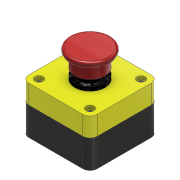
# Autodesk Inventor part: E-Stop
Saved by Autodesk Inventor 2022 (Build 260153000, 153)
## iProperties
Created: 2016-03-20
Part Number: E-Stop
Material: Generic
Document SubType Name: Modeling
Designer: Administrator
Density: 1 g/cm^3
Appearance: Default
Author: Administrator
Autodesk Inventor part; units mm, degrees
ref_plane "YZ Plane" through (0, 0, 0) normal (1, 0, 0) x (0, 1, 0)
ref_plane "XZ Plane" through (0, 0, 0) normal (0, 1, 0) x (-1, 0, 0)
ref_plane "XY Plane" through (0, 0, 0) normal (0, 0, 1) x (1, 0, 0)
sketch "Sketch1" plane through (0, 0, 0) normal (0, 0, 1) x (1, 0, 0)
  line L0 (-34, 34) -> (34, 34)
  line L1 (34, 34) -> (34, -34)
  line L2 (34, -34) -> (-34, -34)
  line L3 (-34, -34) -> (-34, 34)
  point P0 (0, 0)
  dimension "d0" = 34
  dimension "d1" = 34
  dimension "d2" = 34
  dimension "d3" = 34
  constraints: 8 end point, 2 parallel, 1 horizontal, 1 perpendicular
  measures "d0" distance from line of L3 point (0, 0)
  measures "d1" distance from line of L2 point (0, 0)
  measures "d2" distance from line of L1 point (0, 0)
  measures "d3" distance from line of L0 point (0, 0)
extrude "Extrusion1" add sketch "Sketch1" along normal blind 19
sketch "Sketch2" plane through (0, 0, 19) normal (0, 0, 1) x (1, 0, 0)
  circle A0 centre (0, 0) radius 15
  dimension "d6" = 30
  constraints: 1 centre point, 1 coincident
  measures "d6" diameter of A0
extrude "Extrusion2" add sketch "Sketch2" along normal blind 4
sketch "Sketch3" plane through (0, 0, 23) normal (0, 0, 1) x (1, 0, 0)
  circle A0 centre (0, 0) radius 11.25
  dimension "d9" = 22.5
  constraints: 1 centre point, 1 coincident
  measures "d9" diameter of A0
extrude "Extrusion3" add sketch "Sketch3" along normal blind 6
sketch "Sketch4" plane through (0, 0, 29) normal (0, 0, 1) x (1, 0, 0)
  circle A0 centre (0, 0) radius 15
  dimension "d12" = 30
  constraints: 1 centre point, 1 coincident
  measures "d12" diameter of A0
extrude "Extrusion4" add sketch "Sketch4" along normal blind 12
sketch "Sketch5" plane through (0, 0, 41) normal (0, 0, 1) x (1, 0, 0)
  circle A0 centre (0, 0) radius 20
  dimension "d15" = 40
  constraints: 1 centre point, 1 coincident
  measures "d15" diameter of A0
extrude "Extrusion5" add sketch "Sketch5" along normal blind 6
fillet "Fillet1" radius 2 1 edges at (-20, 0, 47)
fillet "Fillet2" radius 3 1 edges at (-20, 0, 41)
fillet "Fillet3" radius 7 4 edges at (34, 34, 9.5) (-34, 34, 9.5) (34, -34, 9.5) (-34, -34, 9.5)
sketch "Sketch6" plane through (0, 0, 0) normal (0, 0, -1) x (-1, 0, 0)
  arc A0 (-27, 34) -> (-34, 27) centre (-27, 27) ccw projected
  arc A1 (27, -34) -> (34, -27) centre (27, -27) ccw projected
  line L0 (-27, 27) -> (27, -27)
  arc A2 (34, 27) -> (27, 34) centre (27, 27) ccw projected
  arc A3 (-34, -27) -> (-27, -34) centre (-27, -27) ccw projected
  line L1 (27, 27) -> (-27, -27)
  circle A4 centre (-25.4, 25.4) radius 2.5
  circle A5 centre (25.4, 25.4) radius 2.5
  circle A6 centre (25.4, -25.4) radius 2.5
  circle A7 centre (-25.4, -25.4) radius 2.5
  point P0 (0, 0)
  dimension "d21" = 5
  dimension "d22" = 25.4
  dimension "d23" = 5
  dimension "d24" = 5
  dimension "d25" = 5
  constraints: 4 centre point, 4 end point, 4 point on line
  measures "d21" diameter of A4
  measures "d22" horizontal distance of point (0, 0) A4.centre
  measures "d23" diameter of A5
  measures "d24" diameter of A6
  measures "d25" diameter of A7
extrude "Extrusion6" cut sketch "Sketch6" against normal blind 20
sketch "Sketch7" plane through (0, 0, 19) normal (0, 0, 1) x (1, 0, 0)
  circle A0 centre (-25.4, 25.4) radius 2.5 projected
  circle A1 centre (-25.4, 25.4) radius 4
  circle A2 centre (25.4, 25.4) radius 2.5 projected
  circle A3 centre (25.4, 25.4) radius 4
  circle A4 centre (25.4, -25.4) radius 2.5 projected
  circle A5 centre (25.4, -25.4) radius 4
  circle A6 centre (-25.4, -25.4) radius 2.5 projected
  circle A7 centre (-25.4, -25.4) radius 4
  point P0 (0, 0)
  dimension "d28" = 8
  dimension "d29" = 8
  dimension "d30" = 8
  dimension "d31" = 8
  constraints: 4 centre point, 4 coincident
  measures "d28" diameter of A1
  measures "d29" diameter of A3
  measures "d30" diameter of A5
  measures "d31" diameter of A7
extrude "Extrusion7" cut sketch "Sketch7" against normal blind 3
sketch "Sketch8" plane through (0, 0, 0) normal (0, 0, -1) x (-1, 0, 0)
  line L0 (-13, 29) -> (13, 29)
  line L1 (18, 24) -> (18, -24)
  line L2 (13, -29) -> (-13, -29)
  line L3 (-18, -24) -> (-18, 24)
  arc A0 (-13, 29) -> (-18, 24) centre (-13, 24) ccw
  arc A1 (18, 24) -> (13, 29) centre (13, 24) ccw
  arc A2 (13, -29) -> (18, -24) centre (13, -24) ccw
  arc A3 (-18, -24) -> (-13, -29) centre (-13, -24) ccw
  point P0 (0, 0)
  dimension "d34" = 18
  dimension "d35" = 18
  dimension "d36" = 29
  dimension "d37" = 29
  dimension "d38" = 5
  constraints: 8 end point, 8 point on circle, 8 tangent, 4 centre point, 3 equal radius, 2 parallel, 1 horizontal, 1 perpendicular
  measures "d34" distance from line of L3 point (0, 0)
  measures "d35" distance from line of L1 point (0, 0)
  measures "d36" distance from line of point (0, 0) L0
  measures "d37" distance from line of L2 point (0, 0)
  measures "d38" radius of A0
extrude "Extrusion8" add sketch "Sketch8" along normal blind 25
sketch "Sketch9" plane through (0, 0, 0) normal (0, 0, -1) x (-1, 0, 0)
  arc A0 (18, 24) -> (13, 29) centre (13, 24) ccw projected
  line L0 (18, 24) -> (18, -24) projected
  arc A1 (13, -29) -> (18, -24) centre (13, -24) ccw projected
  line L1 (13, -29) -> (-13, -29) projected
  arc A2 (-18, -24) -> (-13, -29) centre (-13, -24) ccw projected
  line L2 (-18, -24) -> (-18, 24) projected
  arc A3 (-13, 29) -> (-18, 24) centre (-13, 24) ccw projected
  line L3 (-13, 29) -> (13, 29) projected
  circle A4 centre (25.4, -25.4) radius 2.5 projected
  circle A5 centre (-25.4, 25.4) radius 2.5 projected
  circle A6 centre (25.4, 25.4) radius 2.5 projected
  circle A7 centre (-25.4, -25.4) radius 2.5 projected
  arc A8 (27, -34) -> (34, -27) centre (27, -27) ccw projected
  line L4 (34, -27) -> (34, 27) projected
  arc A9 (34, 27) -> (27, 34) centre (27, 27) ccw projected
  line L5 (27, 34) -> (-27, 34) projected
  arc A10 (-27, 34) -> (-34, 27) centre (-27, 27) ccw projected
  line L6 (-34, 27) -> (-34, -27) projected
  arc A11 (-34, -27) -> (-27, -34) centre (-27, -27) ccw projected
  line L7 (-27, -34) -> (27, -34) projected
  line L8 (-34, 27) -> (-34, -27) projected
  arc A12 (-27, 34) -> (-34, 27) centre (-27, 27) ccw projected
  line L9 (-34, -27) -> (-34, 27)
  line L10 (-27, 34) -> (27, 34)
  arc A13 (27, -34) -> (34, -27) centre (27, -27) ccw projected
  line L11 (34, 27) -> (34, -27)
  line L12 (27, -34) -> (-27, -34)
  arc A14 (-34, -27) -> (-27, -34) centre (-27, -27) ccw
  arc A15 (-27, 34) -> (-34, 27) centre (-27, 27) ccw
  line L13 (-27, 34) -> (27, 34) projected
  arc A16 (34, 27) -> (27, 34) centre (27, 27) ccw
  arc A17 (27, -34) -> (34, -27) centre (27, -27) ccw
  line L14 (-30.6, -24.3) -> (-30.6, 24.3)
  line L15 (-24.3, 30.6) -> (24.3, 30.6)
  line L16 (30.6, 24.3) -> (30.6, -24.3)
  line L17 (24.3, -30.6) -> (-24.3, -30.6)
  arc A18 (-30.6, -24.3) -> (-24.3, -30.6) centre (-24.3, -24.3) ccw
  arc A19 (-24.3, 30.6) -> (-30.6, 24.3) centre (-24.3, 24.3) ccw
  arc A20 (30.6, 24.3) -> (24.3, 30.6) centre (24.3, 24.3) ccw
  arc A21 (24.3, -30.6) -> (30.6, -24.3) centre (24.3, -24.3) ccw
  point P0 (0, 0)
  point P1 (0, 0)
  constraints: 17 point on circle, 16 end point, 8 centre point, 5 tangent, 4 vertical, 2 horizontal, 1 collinear, 1 concentric
extrude "Extrusion9" add sketch "Sketch9" along normal up to surface (25 mm away) separate body contours L7 A11 L6 A10 L5 A9 L4 A8
sketch "Sketch10" plane through (-34, -27, 0) normal (-1, 0, 0) x (0, 0, 1)
  circle A0 centre (-13.2898, 27) radius 5
  point P0 (0, 27)
  dimension "d43" = 10
  constraints: 1 centre point
  measures "d43" diameter of A0
extrude "Extrusion10" cut sketch "Sketch10" against normal blind 10 bodies 2
sketch "Sketch11" plane through (27, -34, -25) normal (0, 0, -1) x (-1, 0, 0)
  arc A0 (-3.6, 9.7) -> (2.7, 3.4) centre (2.7, 9.7) ccw projected
  line L0 (-3.6, 9.7) -> (-3.6, 58.3) projected
  arc A1 (2.7, 64.6) -> (-3.6, 58.3) centre (2.7, 58.3) ccw projected
  line L1 (2.7, 64.6) -> (51.3, 64.6) projected
  arc A2 (57.6, 58.3) -> (51.3, 64.6) centre (51.3, 58.3) ccw projected
  line L2 (57.6, 58.3) -> (57.6, 9.7) projected
  arc A3 (51.3, 3.4) -> (57.6, 9.7) centre (51.3, 9.7) ccw projected
  line L3 (51.3, 3.4) -> (2.7, 3.4) projected
  line L4 (0, 0) -> (54, 0) projected
  arc A4 (54, 0) -> (61, 7) centre (54, 7) ccw projected
  line L5 (61, 7) -> (61, 61) projected
  arc A5 (61, 61) -> (54, 68) centre (54, 61) ccw projected
  line L6 (54, 68) -> (0, 68) projected
  arc A6 (0, 68) -> (-7, 61) centre (0, 61) ccw projected
  line L7 (-7, 61) -> (-7, 7) projected
  arc A7 (-7, 7) -> (0, 0) centre (0, 7) ccw projected
  point P0 (27, 34)
extrude "Extrusion11" add sketch "Sketch11" along normal blind 3 contours L0 A1 L1 A2 L2 A3 L3 A0 | A7 L7 A6 L6 A5 L5 A4 L4 bodies 2
body "Solid1"
body "Solid2"
